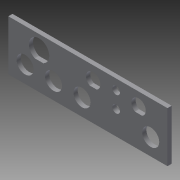
# Autodesk Inventor part: DishFront_BackPlate
Saved by Autodesk Inventor 2014 (Build 180170000, 170)
## iProperties
Created: 2015-01-07
Part Number: DishFront_BackPlate
Material: Generic
Document SubType Name: Modeling
Designer: Owner
Density: 1 g/cm^3
Appearance: Default
Author: Owner
Autodesk Inventor part; units mm, degrees
ref_plane "YZ Plane" through (0, 0, 0) normal (1, 0, 0) x (0, 1, 0)
ref_plane "XZ Plane" through (0, 0, 0) normal (0, 1, 0) x (-1, 0, 0)
ref_plane "XY Plane" through (0, 0, 0) normal (0, 0, 1) x (1, 0, 0)
sketch "Sketch1" plane through (0, 0, 0) normal (0, 0, 1) x (1, 0, 0)
  line L0 (-131.3923, -13.6452) -> (-10.7423, -13.6452)
  line L1 (-10.7423, -13.6452) -> (-10.7423, -51.7452)
  line L2 (-10.7423, -51.7452) -> (-131.3923, -51.7452)
  line L3 (-131.3923, -51.7452) -> (-131.3923, -13.6452)
  point P0 (0, 0)
  dimension "d0" = 120.65
  dimension "d1" = 38.1
  constraints: 8 end point, 2 parallel, 1 horizontal, 1 perpendicular
  measures "d0" distance of L0.start L0.end
  measures "d1" distance of L0.end L1.end
extrude "Extrusion1" add sketch "Sketch1" along normal blind 3.175
sketch "Sketch2" plane through (0, 0, 3.175) normal (0, 0, 1) x (1, 0, 0)
  line L0 (-131.3923, -13.6452) -> (-131.3923, -51.7452) projected
  line L1 (-131.3923, -51.7452) -> (-10.7423, -51.7452) projected
  line L2 (-10.7423, -51.7452) -> (-10.7423, -13.6452) projected
  circle A0 centre (-118.6923, -39.0452) radius 6.477
  circle A1 centre (-23.4423, -39.0452) radius 6.477
  circle A2 centre (-97.1023, -39.0452) radius 6.477
  circle A3 centre (-75.5123, -39.0452) radius 6.477
  line L3 (-10.7423, -13.6452) -> (-131.3923, -13.6452) projected
  circle A4 centre (-108.1143, -24.2104) radius 10.3124 construction
  arc A5 (-104.8718, -31.2462) -> (-111.3567, -31.2462) centre (-108.1143, -24.2104) ccw
  circle A6 centre (-67.0291, -23.5507) radius 9.0932 construction
  arc A7 (-64.29, -28.2751) -> (-69.7682, -28.2751) centre (-67.0291, -23.5507) ccw
  circle A8 centre (-49.6427, -21.3902) radius 5.2451 construction
  circle A9 centre (-49.6427, -21.3902) radius 2.9464
  line L4 (-111.3567, -31.2462) -> (-104.8718, -31.2462)
  line L5 (-69.7682, -28.2751) -> (-64.29, -28.2751)
  circle A10 centre (-32.6262, -23.5507) radius 9.0932 construction
  arc A11 (-29.8871, -28.2751) -> (-35.3653, -28.2751) centre (-32.6262, -23.5507) ccw
  line L6 (-35.3653, -28.2751) -> (-29.8871, -28.2751)
  circle A12 centre (-49.6427, -33.6386) radius 5.2451 construction
  circle A13 centre (-49.6427, -33.6386) radius 2.9464
  point P0 (0, 0)
  dimension "d4" = 12.954
  dimension "d5" = 12.954
  dimension "d6" = 12.954
  dimension "d7" = 12.954
  dimension "d8" = 12.7
  dimension "d9" = 12.7
  dimension "d10" = 12.7
  dimension "d11" = 12.7
  dimension "d12" = 12.7
  dimension "d13" = 12.7
  dimension "d14" = 21.59
  dimension "d15" = 21.59
  dimension "d18" = 20.6248
  dimension "d19" = 15.494
  dimension "d20" = 18.1864
  dimension "d21" = 10.922
  dimension "d22" = 10.4902
  dimension "d23" = 5.8928
  dimension "d24" = 7.0358
  dimension "d25" = 4.7244
  dimension "d26" = 18.1864
  dimension "d27" = 10.922
  dimension "d28" = 4.7244
  dimension "d29" = 10.4902
  dimension "d30" = 5.8928
  constraints: 14 centre point, 6 end point, 6 point on circle, 5 coincident, 2 parallel
  measures "d4" diameter of A0
  measures "d5" diameter of A2
  measures "d6" diameter of A3
  measures "d7" diameter of A1
  measures "d8" distance from line of L1 A0.centre
  measures "d9" distance from line of L1 A2.centre
  measures "d10" distance from line of L1 A3.centre
  measures "d11" distance from line of L1 A1.centre
  measures "d12" distance from line of L0 A0.centre
  measures "d13" distance from line of L2 A1.centre
  measures "d14" distance of A2.centre A0.centre
  measures "d15" distance of A3.centre A2.centre
  measures "d18" diameter of A4
  measures "d19" diameter of A5
  measures "d20" diameter of A6
  measures "d21" diameter of A7
  measures "d22" diameter of A8
  measures "d23" diameter of A9
  measures "d24" distance from line of L4 A4.centre
  measures "d25" distance from line of L5 A6.centre
  measures "d26" diameter of A10
  measures "d27" diameter of A11
  measures "d28" distance from line of L6 A10.centre
  measures "d29" diameter of A12
  measures "d30" diameter of A13
extrude "Extrusion2" cut sketch "Sketch2" against normal blind 6.35 contours A0 | A1 | A2 | A3 | L4 A5 | L5 A7 | A9 | L6 A11 | A13
body "Solid1"
